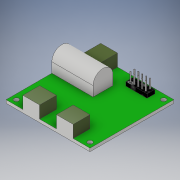
# Autodesk Inventor part: Sterownik-motor
Saved by Autodesk Inventor 2019 (Build 230136000, 136)
## iProperties
Created: 2019-05-01
Part Number: Sterownik-motor
Material: Generic
Document SubType Name: Modeling
Designer: John
Density: 1 g/cm^3
Appearance: Default
Mass: 13.1608 g
Surface Area: 86.3293 cm^2
Volume: 13.1608 cm^3
Author: John
Autodesk Inventor part; units mm, degrees
ref_plane "YZ Plane" through (0, 0, 0) normal (1, 0, 0) x (0, 1, 0)
ref_plane "XZ Plane" through (0, 0, 0) normal (0, 1, 0) x (-1, 0, 0)
ref_plane "XY Plane" through (0, 0, 0) normal (0, 0, 1) x (1, 0, 0)
sketch "Sketch1" plane through (0, 0, 0) normal (0, 1, 0) x (-1, 0, 0)
  line L0 (0, 0) -> (55, 0)
  line L1 (55, 0) -> (55, -55)
  line L2 (55, -55) -> (0, -55)
  line L3 (0, -55) -> (0, 0)
  line L4 (0, 0) -> (3.4, 0)
  line L5 (0, -3.4) -> (0, 0)
  line L6 (55, -55) -> (51.6, -55)
  line L7 (55, -51.6) -> (55, -55)
  circle A0 centre (3.4, -3.4) radius 1.5
  circle A1 centre (51.6, -51.6) radius 1.5
  circle A2 centre (51.6, -3.4) radius 1.5
  circle A3 centre (3.4, -51.6) radius 1.5
  line L8 (0, -55) -> (16.6, -55)
  line L9 (16.6, -55) -> (16.6, -47)
  line L10 (16.6, -47) -> (16.6, -52)
  line L11 (16.6, -47) -> (23.6, -47)
  line L12 (23.6, -47) -> (23.6, -52)
  line L13 (23.6, -52) -> (16.6, -52)
  line L14 (16.6, -52) -> (16.6, -47)
  line L15 (16.6, -52) -> (9.6, -52)
  line L16 (9.6, -52) -> (9.6, -47)
  line L17 (9.6, -47) -> (16.6, -47)
  line L18 (16.6, -47) -> (16.6, -52)
  dimension "d0" = 55
  dimension "d1" = 55
  dimension "d6" = 3
  dimension "d7" = 3
  dimension "d8" = 3
  dimension "d9" = 3
  dimension "d10" = 16.6
  dimension "d11" = 8
  dimension "d12" = 5
  dimension "d13" = 7
  dimension "d14" = 5
  dimension "d15" = 7
  dimension "d16" = 5
  constraints: 38 end point, 6 parallel, 5 horizontal, 4 centre point, 4 perpendicular, 2 point on line
  measures "d0" distance of L1.end L2.end
  measures "d1" distance of L0.end L1.end
  measures "d6" diameter of A0
  measures "d7" diameter of A1
  measures "d8" diameter of A2
  measures "d9" diameter of A3
  measures "d10" distance of L2.end L8.end
  measures "d11" distance of L8.end L9.end
  measures "d12" distance of L9.end L10.end
  measures "d13" distance of L12.end L13.end
  measures "d14" distance of L11.end L12.end
  measures "d15" distance of L16.end L17.end
  measures "d16" distance of L15.end L16.end
extrude "Extrusion1" add sketch "Sketch1" along normal blind 2
sketch "Sketch2" plane through (0, 2, 0) normal (0, 1, 0) x (1, 0, 0)
  line L0 (-55, 0) -> (-44, 0)
  line L1 (-55, 0) -> (0, 0) projected
  line L2 (-44, 10) -> (-44, 0)
  line L3 (0, 0) -> (0, 55) projected
  line L4 (0, 0) -> (-11, 0)
  line L5 (-11, 10) -> (-11, 0)
  line L6 (-44, 0) -> (-33, 0)
  line L7 (-33, 0) -> (-33, 11)
  line L8 (-33, 11) -> (-44, 11)
  line L9 (-44, 11) -> (-44, 0)
  line L10 (-11, 0) -> (-22, 0)
  line L11 (-22, 0) -> (-22, 11)
  line L12 (-22, 11) -> (-11, 11)
  line L13 (-11, 11) -> (-11, 0)
  dimension "d19" = 11
  dimension "d22" = 11
  dimension "d25" = 11
  dimension "d26" = 11
  dimension "d27" = 11
  dimension "d28" = 11
  constraints: 24 end point, 4 parallel, 2 horizontal, 2 perpendicular, 2 point on line
  measures "d19" distance of L0.start L0.end
  measures "d22" distance of L1.end L4.end
  measures "d25" distance of L8.end L7.end
  measures "d26" distance of L7.end L6.end
  measures "d27" distance of L11.end L12.end
  measures "d28" distance of L10.end L11.end
extrude "Extrusion2" add sketch "Sketch2" along normal blind 8
sketch "Sketch3" plane through (0, 2, 0) normal (0, 1, 0) x (1, 0, 0)
  line L0 (-55, 55) -> (-55, 0) projected
  line L1 (-55, 55) -> (-48, 55)
  line L2 (0, 55) -> (-55, 55) projected
  line L3 (-48, 55) -> (-37, 55)
  line L4 (-37, 55) -> (-37, 44)
  line L5 (-37, 44) -> (-48, 44)
  line L6 (-48, 44) -> (-48, 55)
  point P0 (0, 0)
  dimension "d31" = 7
  dimension "d32" = 11
  dimension "d33" = 11
  constraints: 10 end point, 2 parallel, 1 horizontal, 1 perpendicular, 1 point on line
  measures "d31" distance of L0.start L1.end
  measures "d32" distance of L4.end L5.end
  measures "d33" distance of L3.end L4.end
extrude "Extrusion3" add sketch "Sketch3" along normal blind 8
sketch "Sketch4" plane through (0, 2, 0) normal (0, 1, 0) x (1, 0, 0)
  line L0 (-55, 55) -> (-55, 0) projected
  line L1 (-55, 55) -> (-55, 43)
  line L2 (-55, 43) -> (-28, 43)
  line L3 (-28, 43) -> (-28, 30)
  line L4 (-28, 30) -> (-55, 30)
  line L5 (-55, 30) -> (-55, 43)
  point P0 (0, 0)
  dimension "d36" = 12
  dimension "d37" = 27
  dimension "d38" = 13
  constraints: 10 end point, 2 parallel, 1 horizontal, 1 perpendicular, 1 point on line
  measures "d36" distance of L0.start L1.end
  measures "d37" distance of L3.end L4.end
  measures "d38" distance of L2.end L3.end
extrude "Extrusion4" add sketch "Sketch4" along normal blind 13
fillet "Fillet1" radius 6.5 2 edges at (-41.5, 15, -30) (-41.5, 15, -43)
sketch "Sketch5" plane through (0, 2, 0) normal (0, 1, 0) x (1, 0, 0)
  line L0 (-9.6, 47) -> (-23.6, 47) projected
  line L1 (-23.6, 52) -> (-9.6, 52) projected
  line L2 (-9.6, 47) -> (-23.6, 47)
  line L3 (-23.6, 47) -> (-23.6, 52)
  line L4 (-23.6, 52) -> (-9.6, 52)
  line L5 (-9.6, 52) -> (-9.6, 47)
  line L6 (-16.6, 49.5) -> (-16.6, 48.23)
  line L7 (-16.6, 48.23) -> (-19.14, 48.23)
  line L8 (-19.14, 48.23) -> (-21.68, 48.23)
  line L9 (-16.6, 48.23) -> (-14.06, 48.23)
  line L10 (-14.06, 48.23) -> (-11.52, 48.23)
  line L11 (-11.52, 48.23) -> (-11.52, 50.77)
  line L12 (-11.27, 48.48) -> (-11.77, 48.48)
  line L13 (-11.77, 48.48) -> (-11.77, 47.98)
  line L14 (-11.77, 47.98) -> (-11.27, 47.98)
  line L15 (-11.27, 47.98) -> (-11.27, 48.48)
  line L16 (-11.27, 48.48) -> (-11.77, 47.98) construction
  line L17 (-11.77, 48.48) -> (-11.27, 47.98) construction
  line L18 (-13.81, 48.48) -> (-14.31, 48.48)
  line L19 (-14.31, 48.48) -> (-14.31, 47.98)
  line L20 (-14.31, 47.98) -> (-13.81, 47.98)
  line L21 (-13.81, 47.98) -> (-13.81, 48.48)
  line L22 (-13.81, 48.48) -> (-14.31, 47.98) construction
  line L23 (-14.31, 48.48) -> (-13.81, 47.98) construction
  line L24 (-16.35, 48.48) -> (-16.85, 48.48)
  line L25 (-16.85, 48.48) -> (-16.85, 47.98)
  line L26 (-16.85, 47.98) -> (-16.35, 47.98)
  line L27 (-16.35, 47.98) -> (-16.35, 48.48)
  line L28 (-16.35, 48.48) -> (-16.85, 47.98) construction
  line L29 (-16.85, 48.48) -> (-16.35, 47.98) construction
  line L30 (-18.89, 48.48) -> (-19.39, 48.48)
  line L31 (-19.39, 48.48) -> (-19.39, 47.98)
  line L32 (-19.39, 47.98) -> (-18.89, 47.98)
  line L33 (-18.89, 47.98) -> (-18.89, 48.48)
  line L34 (-18.89, 48.48) -> (-19.39, 47.98) construction
  line L35 (-19.39, 48.48) -> (-18.89, 47.98) construction
  line L36 (-21.93, 48.48) -> (-21.43, 48.48)
  line L37 (-21.43, 48.48) -> (-21.43, 47.98)
  line L38 (-21.43, 47.98) -> (-21.93, 47.98)
  line L39 (-21.93, 47.98) -> (-21.93, 48.48)
  line L40 (-21.93, 48.48) -> (-21.43, 47.98) construction
  line L41 (-21.43, 48.48) -> (-21.93, 47.98) construction
  line L42 (-11.27, 51.02) -> (-11.77, 51.02)
  line L43 (-11.77, 51.02) -> (-11.77, 50.52)
  line L44 (-11.77, 50.52) -> (-11.27, 50.52)
  line L45 (-11.27, 50.52) -> (-11.27, 51.02)
  line L46 (-11.27, 51.02) -> (-11.77, 50.52) construction
  line L47 (-11.77, 51.02) -> (-11.27, 50.52) construction
  line L48 (-13.75, 51.02) -> (-14.25, 51.02)
  line L49 (-14.25, 51.02) -> (-14.25, 50.52)
  line L50 (-14.25, 50.52) -> (-13.75, 50.52)
  line L51 (-13.75, 50.52) -> (-13.75, 51.02)
  line L52 (-13.75, 51.02) -> (-14.25, 50.52) construction
  line L53 (-14.25, 51.02) -> (-13.75, 50.52) construction
  line L54 (-16.35, 50.52) -> (-16.85, 50.52)
  line L55 (-16.85, 50.52) -> (-16.85, 51.02)
  line L56 (-16.85, 51.02) -> (-16.35, 51.02)
  line L57 (-16.35, 51.02) -> (-16.35, 50.52)
  line L58 (-16.35, 50.52) -> (-16.85, 51.02) construction
  line L59 (-16.85, 50.52) -> (-16.35, 51.02) construction
  line L60 (-18.89, 50.52) -> (-19.39, 50.52)
  line L61 (-19.39, 50.52) -> (-19.39, 51.02)
  line L62 (-19.39, 51.02) -> (-18.89, 51.02)
  line L63 (-18.89, 51.02) -> (-18.89, 50.52)
  line L64 (-18.89, 50.52) -> (-19.39, 51.02) construction
  line L65 (-19.39, 50.52) -> (-18.89, 51.02) construction
  line L66 (-21.43, 50.52) -> (-21.93, 50.52)
  line L67 (-21.93, 50.52) -> (-21.93, 51.02)
  line L68 (-21.93, 51.02) -> (-21.43, 51.02)
  line L69 (-21.43, 51.02) -> (-21.43, 50.52)
  line L70 (-21.43, 50.52) -> (-21.93, 51.02) construction
  line L71 (-21.93, 50.52) -> (-21.43, 51.02) construction
  point P0 (0, 0)
  point P1 (-14, 50.77)
  point P2 (-16.6, 50.77)
  point P3 (-19.14, 50.77)
  point P4 (-21.68, 50.77)
  dimension "d42" = 1.27
  dimension "d43" = 2.54
  dimension "d44" = 2.54
  dimension "d45" = 2.54
  dimension "d46" = 2.54
  dimension "d47" = 2.54
  dimension "d48" = 0.5
  dimension "d49" = 0.5
  dimension "d50" = 0.5
  dimension "d51" = 0.5
  dimension "d52" = 0.5
  dimension "d53" = 0.5
  dimension "d54" = 0.5
  dimension "d55" = 0.5
  dimension "d56" = 0.5
  dimension "d57" = 0.5
  dimension "d58" = 0.5
  dimension "d59" = 0.5
  constraints: 140 end point, 22 parallel, 20 midpoint, 13 perpendicular, 12 horizontal, 3 point on line, 1 vertical
  measures "d42" distance of L6.start L6.end
  measures "d43" distance of L6.end L7.end
  measures "d44" distance of L7.end L8.end
  measures "d45" distance of L6.end L9.end
  measures "d46" distance of L9.end L10.end
  measures "d47" distance of L10.end L11.end
  measures "d48" distance of L14.end L13.end
  measures "d49" distance of L13.end L12.end
  measures "d50" distance of L20.end L19.end
  measures "d51" distance of L26.end L25.end
  measures "d52" distance of L25.end L24.end
  measures "d53" distance of L32.end L31.end
  measures "d54" distance of L31.end L30.end
  measures "d55" distance of L37.end L38.end
  measures "d56" distance of L36.end L37.end
  measures "d57" distance of L44.end L43.end
  measures "d58" distance of L43.end L42.end
  measures "d59" distance of L50.end L49.end
extrude "Extrusion5" add sketch "Sketch5" along normal blind 8.5 contours L24 L27 L9 L6 | L6 L7 L25 L24 | L9 L27 L26 L25 L7 | L33 L32 L31 L8 L7 | L7 L8 L31 L30 L33 | L19 L18 L21 L10 L9 | L9 L10 L21 L20 L19 | L13 L12 L11 L10 | L10 L11 L12 L15 L14 L13 | L36 L37 L38 L39 | L45 L44 L43 L42 | L51 L50 L49 L48 | L54 L55 L56 L57 | L60 L61 L62 L63 | L66 L67 L68 L69
sketch "Sketch6" plane through (0, 2, 0) normal (0, 1, 0) x (1, 0, 0)
  line L0 (-9.6, 47) -> (-23.6, 47) projected
  line L1 (-23.6, 52) -> (-9.6, 52) projected
  line L2 (-9.6, 47) -> (-23.6, 47)
  line L3 (-23.6, 47) -> (-23.6, 52)
  line L4 (-23.6, 52) -> (-9.6, 52)
  line L5 (-9.6, 52) -> (-9.6, 47)
  point P0 (0, 0)
  constraints: 8 end point, 2 parallel, 1 horizontal, 1 perpendicular
extrude "Extrusion6" add sketch "Sketch6" along normal blind 2.5 and the other way blind 2
body "Solid1"
